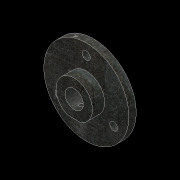
# Autodesk Inventor part: Matrizenhalterung_unten
Saved by Autodesk Inventor 2019 (Build 230136000, 136)
## iProperties
Created: 2022-01-12
Part Number: Matrizenhalterung_unten
Material: Stahl
Document SubType Name: Modeling
Designer: Jonas Nebl
Density: 7.85 g/cm^3
Appearance: Platte
Mass: 250.476 g
Surface Area: 119.902 cm^2
Volume: 31.9077 cm^3
Author: Jonas Nebl
Autodesk Inventor part; units mm, degrees
ref_plane "YZ Plane" through (0, 0, 0) normal (1, 0, 0) x (0, 1, 0)
ref_plane "XY Plane" through (0, 0, 0) normal (0, 0, 1) x (1, 0, 0)
sketch "Skizze1" plane through (0, 0, 0) normal (0, 1, 0) x (-1, 0, 0)
  line L0 (-15, 16) -> (-7.5, 16)
  line L1 (-7.5, 16) -> (-7.5, -10)
  line L2 (-15, 16) -> (-15, 6)
  line L3 (-15, 6) -> (-35, 6)
  line L4 (-35, 6) -> (-35, 0)
  line L5 (-35, 0) -> (-15, 0)
  line L6 (-15, 0) -> (-15, -10)
  line L7 (0, -15.2) -> (0, 21.2) projected
  line L8 (-7.5, -10) -> (-15, -10)
  point P0 (0, 0)
  dimension "d0" = 30
  dimension "d1" = 15
  dimension "d2" = 70
  dimension "d3" = 6
  dimension "d4" = 10
  dimension "d5" = 10
  constraints: 16 end point, 4 horizontal, 4 vertical, 2 point on line
  measures "d0" diameter of L6 L7
  measures "d1" diameter of L1 L7
  measures "d2" diameter of L4 L7
  measures "d3" distance of L3.end L4.end
  measures "d4" distance of L0.start L2.end
  measures "d5" distance of L5.end L6.end
revolve "Umdrehung1" add sketch "Skizze1" angle 360 about axis through (0, 0, -10) along (0, 0, 1)
ref_plane "Arbeitsebene1" through (0, -16, 0) normal (0, 1, 0) x (-1, 0, 0)
sketch "Skizze2" plane through (0, -16, 0) normal (0, 1, 0) x (-1, 0, 0)
  line L0 (15, 16) -> (-15, 16) projected
  line L1 (15, 6) -> (-15, 6) projected
  line L2 (6, 16) -> (-6, 16)
  line L3 (-6, 16) -> (-6, 6)
  line L4 (-6, 6) -> (6, 6)
  line L5 (6, 6) -> (6, 16)
  line L6 (0, -2.8) -> (0, 16.8) projected
  point P0 (0, 0)
  dimension "d8" = 12
  constraints: 8 end point, 2 parallel, 2 point on line, 1 horizontal, 1 perpendicular, 1 other
  measures "d8" distance between parallel lines of L3 L5
extrude "Extrusion1" cut sketch "Skizze2" along normal blind 2
sketch "Skizze4" plane through (0, -14, 0) normal (0, -1, 0) x (1, 0, 0)
  line L0 (-5.3852, 16) -> (5.3852, 16) projected
  point P0 (0, 0)
  point P1 (-0.0015, 10)
  dimension "d18" = 6
  measures "d18" distance from line of L0 point (-0.002, 10)
hole "Bohrung2" at (-0.0015, -14, 10) direction (0, 1, 0) diameter 3.3 depth 10 tip angle 118
thread "Gewinde1" size "M4x0.7" class "6H" standard "ANSI Metric M Profile" full length
sketch "Skizze6" plane through (0, 0, 6) normal (0, 0, 1) x (1, 0, 0)
  circle A0 centre (0, 0) radius 35 projected
  point P0 (0, 26)
  point P1 (-22.5167, -13)
  point P2 (22.5167, -13)
  dimension "d40" = 26
  dimension "d41" = 0
  dimension "d44" = 360
  constraints: 4 other
  measures "d40" distance of point (0, 26) A0.centre
  measures "d41" horizontal distance of A0.centre point (0, 26)
hole "Bohrung4" at (0, 26, 6) at (-22.5167, -13, 6) at (22.5167, -13, 6) direction (0, 0, -1) diameter 6.5 depth 35 tip angle 118
